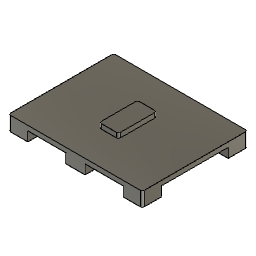
Project Stand Top Plate v9 (Autodesk Fusion 360 design; units mm, degrees)
Autodesk Fusion 360 part; units mm, degrees
sketch "Sketch1" plane through (0, 0, 0) normal (0, 0, 1) x (1, 0, 0)
  line L0 (-75, 55) -> (65.2, 55)
  line L1 (65.2, 55) -> (65.2, -55.2)
  line L2 (65.2, -55.2) -> (-75, -55.2)
  line L3 (-75, -55.2) -> (-75, 55)
  dimension "d1" = 140.2
  dimension "d2" = 110.2
  constraint horizontal L0
  constraint vertical L1
  constraint horizontal L2
  constraint vertical L3
  measures "d1" distance of L0.start L0.end
  measures "d2" distance of L0.end L1.end
extrude "Extrude1" add sketch "Sketch1" along normal blind 5
sketch "Sketch2" plane through (0, 0, 0) normal (0, 0, -1) x (1, 0, 0)
  line L0 (65.2, 55.2) -> (-75, 55.2)
  line L1 (-75, 55.2) -> (-75, -55)
  line L2 (-75, -55) -> (65.2, -55)
  line L3 (65.2, -55) -> (65.2, 55.2)
  line L4 (65.2, -55) -> (45, -55)
  line L5 (45, -55) -> (45, -34.8)
  line L6 (45, -34.8) -> (65.2, -34.8)
  line L7 (65.2, -34.8) -> (65.2, -55)
  line L8 (-75, -55) -> (-54.8, -55)
  line L9 (-54.8, -55) -> (-54.8, -34.8)
  line L10 (-54.8, -34.8) -> (-75, -34.8)
  line L11 (-75, -34.8) -> (-75, -55)
  line L12 (5.2, -55) -> (-15, -55)
  line L13 (-15, -55) -> (-15, -34.8)
  line L14 (-15, -34.8) -> (5.2, -34.8)
  line L15 (5.2, -34.8) -> (5.2, -55)
  line L16 (65.2, 55.2) -> (45, 55.2)
  line L17 (45, 55.2) -> (45, 35)
  line L18 (45, 35) -> (65.2, 35)
  line L19 (65.2, 35) -> (65.2, 55.2)
  line L20 (5.2, 55.2) -> (-15, 55.2)
  line L21 (-15, 55.2) -> (-15, 35)
  line L22 (-15, 35) -> (5.2, 35)
  line L23 (5.2, 35) -> (5.2, 55.2)
  line L24 (-75, 55.2) -> (-54.8, 55.2)
  line L25 (-54.8, 55.2) -> (-54.8, 35)
  line L26 (-54.8, 35) -> (-75, 35)
  line L27 (-75, 35) -> (-75, 55.2)
  line L28 (60.2, -50) -> (50, -50)
  line L29 (50, -50) -> (50, -39.8)
  line L30 (50, -39.8) -> (60.2, -39.8)
  line L31 (60.2, -39.8) -> (60.2, -50)
  line L32 (0.2, -50) -> (-10, -50)
  line L33 (-10, -50) -> (-10, -39.8)
  line L34 (-10, -39.8) -> (0.2, -39.8)
  line L35 (0.2, -39.8) -> (0.2, -50)
  line L36 (-59.8, -50) -> (-70, -50)
  line L37 (-70, -50) -> (-70, -39.8)
  line L38 (-70, -39.8) -> (-59.8, -39.8)
  line L39 (-59.8, -39.8) -> (-59.8, -50)
  line L40 (60.2, 40) -> (50, 40)
  line L41 (50, 40) -> (50, 50.2)
  line L42 (50, 50.2) -> (60.2, 50.2)
  line L43 (60.2, 50.2) -> (60.2, 40)
  line L44 (0.2, 40) -> (-10, 40)
  line L45 (-10, 40) -> (-10, 50.2)
  line L46 (-10, 50.2) -> (0.2, 50.2)
  line L47 (0.2, 50.2) -> (0.2, 40)
  line L48 (-59.8, 40) -> (-70, 40)
  line L49 (-70, 40) -> (-70, 50.2)
  line L50 (-70, 50.2) -> (-59.8, 50.2)
  line L51 (-59.8, 50.2) -> (-59.8, 40)
  dimension "d5" = 20.2
  dimension "d6" = 20.2
  dimension "d7" = 20.2
  dimension "d8" = 39.8
  dimension "d9" = 20.2
  dimension "d10" = 20.2
  dimension "d11" = 39.8
  dimension "d12" = 20.2
  dimension "d13" = 20.2
  dimension "d14" = 20.2
  dimension "d15" = 20.2
  dimension "d16" = 39.8
  dimension "d17" = 20.2
  dimension "d18" = 39.8
  dimension "d19" = 20.2
  dimension "d20" = 20.2
  dimension "d21" = 5
  dimension "d22" = 5
  dimension "d23" = 5
  dimension "d24" = 5
  dimension "d25" = 5
  dimension "d26" = 5
  dimension "d27" = 5
  dimension "d28" = 5
  dimension "d29" = 5
  dimension "d30" = 5
  dimension "d31" = 5
  dimension "d32" = 5
  dimension "d33" = 5
  dimension "d34" = 5
  dimension "d35" = 5
  dimension "d36" = 5
  dimension "d37" = 5
  dimension "d38" = 5
  dimension "d39" = 5
  dimension "d40" = 5
  dimension "d41" = 5
  dimension "d42" = 5
  dimension "d43" = 5
  dimension "d44" = 5
  constraint horizontal L4
  constraint vertical L5
  constraint horizontal L6
  constraint vertical L7
  constraint coincident L2.end L3.start
  constraint horizontal L8
  constraint vertical L9
  constraint horizontal L10
  constraint vertical L11
  constraint coincident L1.end L2.start
  constraint horizontal L12
  constraint vertical L13
  constraint horizontal L14
  constraint vertical L15
  constraint coincident L2 L12.start
  constraint horizontal L16
  constraint vertical L17
  constraint horizontal L18
  constraint vertical L19
  constraint coincident L0.start L3.end
  constraint horizontal L20
  constraint vertical L21
  constraint horizontal L22
  constraint vertical L23
  constraint coincident L0 L20.start
  constraint horizontal L24
  constraint vertical L25
  constraint horizontal L26
  constraint vertical L27
  constraint coincident L0.end L1.start
  constraint horizontal L28
  constraint vertical L29
  constraint horizontal L30
  constraint vertical L31
  constraint horizontal L32
  constraint vertical L33
  constraint horizontal L34
  constraint vertical L35
  constraint horizontal L36
  constraint vertical L37
  constraint horizontal L38
  constraint vertical L39
  constraint horizontal L40
  constraint vertical L41
  constraint horizontal L42
  constraint vertical L43
  constraint horizontal L44
  constraint vertical L45
  constraint horizontal L46
  constraint vertical L47
  constraint horizontal L48
  constraint vertical L49
  constraint horizontal L50
  constraint vertical L51
  measures "d5" distance of L17 L19
  measures "d6" distance of L16 L18
  measures "d7" distance of L20 L22
  measures "d8" distance of L17 L23
  measures "d9" distance of L25 L27
  measures "d10" distance of L24 L26
  measures "d11" distance of L21 L25
  measures "d12" distance of L5 L7
  measures "d13" distance of L4 L6
  measures "d14" distance of L8 L10
  measures "d15" distance of L9 L11
  measures "d16" distance of L9 L13
  measures "d17" distance of L12 L14
  measures "d18" distance of L5 L15
  measures "d19" distance of L13 L15
  measures "d20" distance of L21 L23
  measures "d21" distance of L18 L40
  measures "d22" distance of L19 L43
  measures "d23" distance of L17 L41
  measures "d24" distance of L16 L42
  measures "d25" distance of L20 L46
  measures "d26" distance of L23 L47
  measures "d27" distance of L21 L45
  measures "d28" distance of L22 L44
  measures "d29" distance of L26 L48
  measures "d30" distance of L25 L51
  measures "d31" distance of L27 L49
  measures "d32" distance of L24 L50
  measures "d33" distance of L11 L37
  measures "d34" distance of L8 L36
  measures "d35" distance of L9 L39
  measures "d36" distance of L10 L38
  measures "d37" distance of L13 L33
  measures "d38" distance of L12 L32
  measures "d39" distance of L15 L35
  measures "d40" distance of L14 L34
  measures "d41" distance of L6 L30
  measures "d42" distance of L5 L29
  measures "d43" distance of L4 L28
  measures "d44" distance of L7 L31
extrude "Extrude2" cut sketch "Sketch2" against normal blind 2.5 contours L28 L29 L30 L31 | L32 L33 L34 L35 | L36 L37 L38 L39 | L40 L41 L42 L43 | L44 L45 L46 L47 | L48 L49 L50 L51
extrude "Extrude3" add sketch "Sketch2" along normal blind 10 contours L0 L3 L16 L17 L18 L19 | L0 L20 L21 L22 L23 | L2 L3 L4 L5 L6 L7 | L0 L1 L24 L25 L26 L27 | L2 L12 L13 L14 L15 | L1 L2 L8 L9 L10 L11
sketch "Sketch3" plane through (0, 0, 5) normal (0, 0, 1) x (-1, 0, 0)
  line L0 (75, 55.2) -> (-65.2, 55.2)
  line L1 (-65.2, 55.2) -> (-65.2, -55)
  line L2 (-65.2, -55) -> (75, -55)
  line L3 (75, -55) -> (75, 55.2)
  line L4 (14.9, -19.9) -> (-5.1, -19.9)
  line L5 (-5.1, -19.9) -> (-5.1, 20.1)
  line L6 (-5.1, 20.1) -> (14.9, 20.1)
  line L7 (14.9, 20.1) -> (14.9, -19.9)
  dimension "d49" = 20
  dimension "d50" = 40
  dimension "d51" = 110.2
  dimension "d52" = 140.2
  dimension "d53" = 35.1
  dimension "d54" = 35.1
  dimension "d55" = 60.1
  dimension "d56" = 60.1
  constraint horizontal L4
  constraint vertical L5
  constraint horizontal L6
  constraint vertical L7
  measures "d49" distance of L5 L7
  measures "d50" distance of L4.start L6.end
  measures "d51" distance of L0 L2
  measures "d52" distance of L1 L3
  measures "d53" distance of L2 L4
  measures "d54" distance of L0 L6
  measures "d55" distance of L3 L7
  measures "d56" distance of L1 L5
extrude "Extrude4" add sketch "Sketch3" along normal blind 5 contours L4 L5 L6 L7
fillet "Fillet1" radius 2 4 edges at (-75, -55.2, -2.5) (65.2, -55.2, -2.5) (65.2, 55, -2.5) (-75, 55, -2.5)
fillet "Fillet2" radius 2 4 edges at (5.1, -20.1, 7.5) (-14.9, -20.1, 7.5) (5.1, 19.9, 7.5) (-14.9, 19.9, 7.5)
